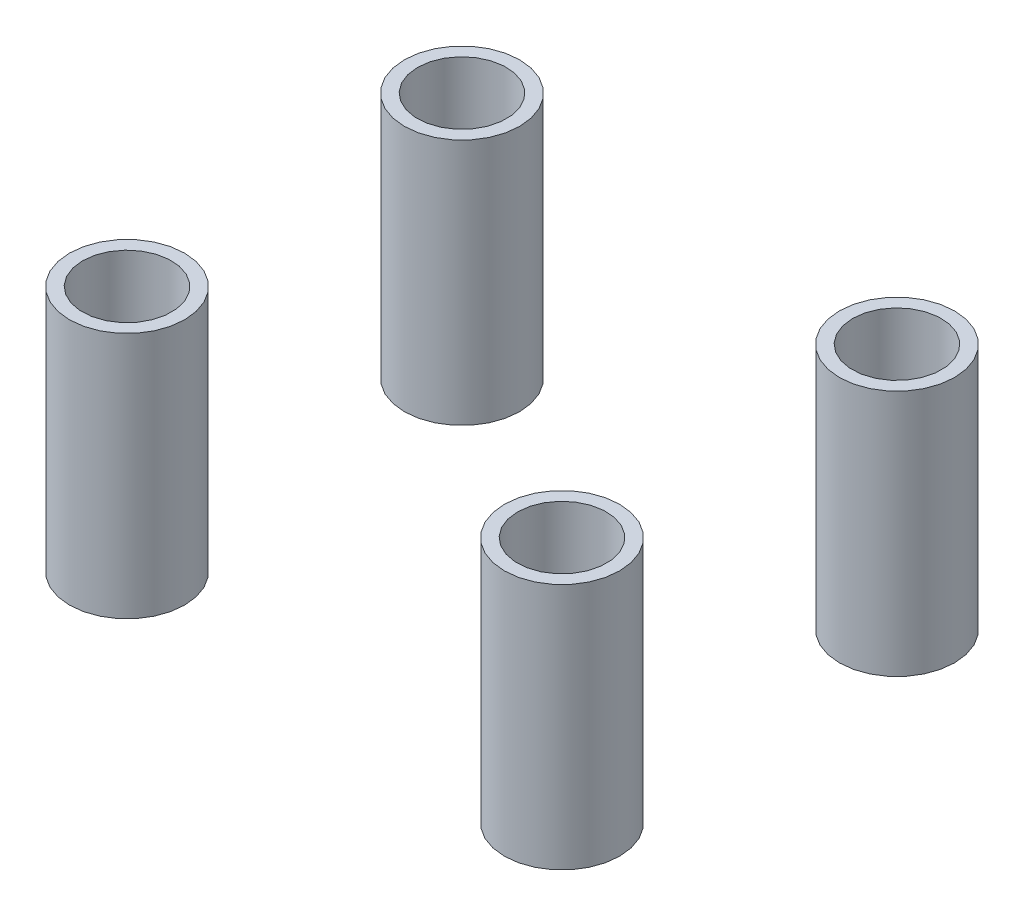
# Autodesk Inventor part: FastenerForLegFrame
Saved by Autodesk Inventor 2027 (Build 310192000, 192)
## iProperties
Created: 2026-07-09
Part Number: FastenerForLegFrame
Material: Generic
Document SubType Name: Modeling
Designer: belcz
Density: 1 g/cm^3
Appearance: Default
Author: belcz
Autodesk Inventor part; units mm, degrees
ref_plane "YZ Plane" through (0, 0, 0) normal (1, 0, 0) x (0, 1, 0)
ref_plane "XZ Plane" through (0, 0, 0) normal (0, 1, 0) x (-1, 0, 0)
ref_plane "XY Plane" through (0, 0, 0) normal (0, 0, 1) x (1, 0, 0)
sketch "Sketch1" plane through (0, 0, 0) normal (0, 1, 0) x (-1, 0, 0)
  arc A0 (17.7231, -22.7881) -> (17.7231, -20.9526) centre (20.7626, -21.8703) ccw projected
  arc A1 (17.7231, -20.9526) -> (17.7231, -22.7881) centre (20.7626, -21.8703) ccw projected
  arc A2 (17.7231, -48.6072) -> (17.7231, -46.7717) centre (20.7626, -47.6894) ccw projected
  arc A3 (17.7231, -46.7717) -> (17.7231, -48.6072) centre (20.7626, -47.6894) ccw projected
  arc A4 (-9.726, -46.7717) -> (-9.726, -48.6072) centre (-12.7654, -47.6894) ccw projected
  arc A5 (-9.726, -48.6072) -> (-9.726, -46.7717) centre (-12.7654, -47.6894) ccw projected
  arc A6 (-9.726, -20.9526) -> (-9.726, -22.7881) centre (-12.7654, -21.8703) ccw projected
  arc A7 (-9.726, -22.7881) -> (-9.726, -20.9526) centre (-12.7654, -21.8703) ccw projected
  circle A8 centre (20.7626, -21.8703) radius 3.429
  circle A9 centre (20.7626, -47.6894) radius 3.429
  circle A10 centre (-12.7654, -47.6894) radius 3.429
  circle A11 centre (-12.7654, -21.8703) radius 3.429
  circle A12 centre (-12.7654, -21.8703) radius 4.445
  circle A13 centre (-12.7654, -47.6894) radius 4.445
  circle A14 centre (20.7626, -47.6894) radius 4.445
  circle A15 centre (20.7626, -21.8703) radius 4.445
  point P0 (0, 0)
  dimension "d0" = 6.858
  dimension "d1" = 6.858
  dimension "d2" = 6.858
  dimension "d3" = 6.858
  dimension "d4" = 8.89
  dimension "d5" = 8.89
  dimension "d6" = 8.89
  dimension "d7" = 8.89
  constraints: 8 centre point, 8 coincident
  measures "d0" diameter of A8
  measures "d1" diameter of A9
  measures "d2" diameter of A10
  measures "d3" diameter of A11
  measures "d4" diameter of A12
  measures "d5" diameter of A13
  measures "d6" diameter of A14
  measures "d7" diameter of A15
extrude "Extrusion1" add sketch "Sketch1" along normal blind 19.05 contours A12 | A13 | A14 | A15
ref_plane "Work Plane2" through (-20.7626, 0, -17.4253) normal (0, 0, 1) x (1, 0, 0)
ref_plane "Work Plane1" through (-4.353, 20.3962, -73.6634) normal (0, 0, 1) x (1, 0, 0)
sketch "Sketch2" plane through (-20.7626, 0, -17.4253) normal (0, 0, 1) x (1, 0, 0)
  line L0 (5.08, 19.05) -> (3.81, 19.05) projected
  line L1 (5.08, 19.1092) -> (6.35, 20.5954) projected
  circle A0 centre (16.4095, 20.3962) radius 7.9375 projected
  line L2 (29.718, 19.05) -> (28.448, 19.05) projected
  line L3 (29.083, 0) -> (29.083, 19.05) projected
  line L4 (29.718, 19.05) -> (37.0078, 19.05) projected
  line L5 (27.178, 20.5954) -> (28.448, 19.1092) projected
  line L6 (28.448, 22.098) -> (28.448, 19.05) projected
  circle A1 centre (16.4095, 20.3962) radius 69.85 projected
  circle A2 centre (16.4095, 20.3962) radius 7.9375 projected
  line L7 (6.35, 20.5954) -> (10.8352, 25.8441) projected
  line L8 (5.08, 19.05) -> (5.08, 22.098) projected
  line L9 (22.6928, 25.8441) -> (27.178, 20.5954) projected
  arc A3 (22.6928, 25.8441) -> (21.7273, 26.289) centre (21.7273, 25.019) ccw projected
  arc A4 (11.8007, 26.289) -> (10.8352, 25.8441) centre (11.8007, 25.019) ccw projected
  point P0 (20.7626, 0)
  constraints: 1 other
body "Solid1"
